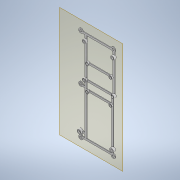
# Autodesk Inventor part: system_holder_plastic
Saved by Autodesk Inventor 2020 (Build 240168000, 168)
## iProperties
Created: 2020-01-14
Part Number: system_holder_plastic
Material: Generic
Document SubType Name: Modeling
Designer: erwin
Density: 1 g/cm^3
Appearance: Default
Author: erwin
Autodesk Inventor part; units mm, degrees
ref_plane "YZ Plane" through (0, 0, 0) normal (1, 0, 0) x (0, 1, 0)
ref_plane "XZ Plane" through (0, 0, 0) normal (0, 1, 0) x (-1, 0, 0)
ref_plane "XY Plane" through (0, 0, 0) normal (0, 0, 1) x (1, 0, 0)
ref_plane "Work Plane1" through (0, 0, 0) normal (0, 0, 1) x (1, 0, 0)
sketch "Sketch1" plane through (0, 0, 0) normal (0, 0, 1) x (1, 0, 0)
  circle A0 centre (-17, 43.4) radius 1.9 projected
  circle A1 centre (-17, 79.8) radius 1.9 projected
  circle A2 centre (39, -79.8) radius 1.9 projected
  circle A3 centre (-17, -79.8) radius 1.9 projected
  circle A4 centre (39, 79.8) radius 1.9 projected
  circle A5 centre (-17, 0) radius 1.9 projected
  circle A6 centre (39, 43.4) radius 1.9 construction
  arc A7 (-25.9799, 38.2) -> (-24, 40.1799) centre (-24.9899, 39.1899) ccw projected
  line L0 (-25.9799, 38.2) -> (-27.6, 38.2) projected
  line L1 (-27.6, 28.2) -> (-27.6, 38.2) projected
  line L2 (-27.6, 28.2) -> (-25.9799, 28.2) projected
  arc A8 (-24, 26.2201) -> (-25.9799, 28.2) centre (-24.9899, 27.2101) ccw projected
  line L3 (-24, 26.2201) -> (-24, 20.1799) projected
  arc A9 (-25.9799, 18.2) -> (-24, 20.1799) centre (-24.9899, 19.1899) ccw projected
  line L4 (-25.9799, 18.2) -> (-27.6, 18.2) projected
  line L5 (-27.6, -18.2) -> (-27.6, 18.2) projected
  line L6 (-27.6, -18.2) -> (-25.9799, -18.2) projected
  arc A10 (-24, -20.1799) -> (-25.9799, -18.2) centre (-24.9899, -19.1899) ccw projected
  line L7 (-24, -20.1799) -> (-24, -26.2201) projected
  arc A11 (-25.9799, -28.2) -> (-24, -26.2201) centre (-24.9899, -27.2101) ccw projected
  line L8 (-25.9799, -28.2) -> (-27.6, -28.2) projected
  line L9 (-27.6, -38.2) -> (-27.6, -28.2) projected
  line L10 (-27.6, -38.2) -> (-25.9799, -38.2) projected
  arc A12 (-24, -40.1799) -> (-25.9799, -38.2) centre (-24.9899, -39.1899) ccw projected
  line L11 (-24, -40.1799) -> (-24, -46.2201) projected
  arc A13 (-25.9799, -48.2) -> (-24, -46.2201) centre (-24.9899, -47.2101) ccw projected
  line L12 (-25.9799, -48.2) -> (-27.6, -48.2) projected
  line L13 (-27.6, -54.6) -> (-27.6, -48.2) projected
  line L14 (-36.9959, -54.6) -> (-27.6, -54.6) projected
  line L15 (-36.9945, -55.6) -> (-36.9959, -54.6) projected
  line L16 (-40.9945, -55.6) -> (-36.9945, -55.6) projected
  line L17 (-40.9959, -54.6) -> (-40.9945, -55.6) projected
  line L18 (-42.6, -54.6) -> (-40.9959, -54.6) projected
  arc A14 (-42.6, -54.6) -> (-42.6, -68.6) centre (-42.6, -61.6) ccw projected
  line L19 (-40.9761, -68.6) -> (-42.6, -68.6) projected
  line L20 (-40.9736, -67.6) -> (-40.9761, -68.6) projected
  line L21 (-36.9736, -67.6) -> (-40.9736, -67.6) projected
  line L22 (-36.9761, -68.6) -> (-36.9736, -67.6) projected
  line L23 (-27.6, -68.6) -> (-36.9761, -68.6) projected
  line L24 (-27.6, -75) -> (-27.6, -68.6) projected
  line L25 (-27.6, -75) -> (-25.9799, -75) projected
  arc A15 (-24, -76.9799) -> (-25.9799, -75) centre (-24.9899, -75.9899) ccw projected
  line L26 (-24, -76.9799) -> (-24, -86.8) projected
  line L27 (-24, -86.8) -> (46, -86.8) projected
  line L28 (46, -86.8) -> (46, -76.9799) projected
  arc A16 (47.9799, -75) -> (46, -76.9799) centre (46.9899, -75.9899) ccw projected
  line L29 (47.9799, -75) -> (49.6, -75) projected
  line L30 (49.6, -48.2) -> (49.6, -75) projected
  line L31 (49.6, -48.2) -> (47.9799, -48.2) projected
  arc A17 (46, -46.2201) -> (47.9799, -48.2) centre (46.9899, -47.2101) ccw projected
  line L32 (46, -46.2201) -> (46, -40.1799) projected
  arc A18 (47.9799, -38.2) -> (46, -40.1799) centre (46.9899, -39.1899) ccw projected
  line L33 (47.9799, -38.2) -> (49.6, -38.2) projected
  line L34 (49.6, -28.2) -> (49.6, -38.2) projected
  line L35 (49.6, -28.2) -> (47.9799, -28.2) projected
  arc A19 (46, -26.2201) -> (47.9799, -28.2) centre (46.9899, -27.2101) ccw projected
  line L36 (46, -26.2201) -> (46, -20.1799) projected
  arc A20 (47.9799, -18.2) -> (46, -20.1799) centre (46.9899, -19.1899) ccw projected
  line L37 (47.9799, -18.2) -> (49.6, -18.2) projected
  line L38 (49.6, 18.2) -> (49.6, -18.2) projected
  line L39 (49.6, 18.2) -> (47.9799, 18.2) projected
  arc A21 (46, 20.1799) -> (47.9799, 18.2) centre (46.9899, 19.1899) ccw projected
  line L40 (46, 20.1799) -> (46, 26.2201) projected
  arc A22 (47.9799, 28.2) -> (46, 26.2201) centre (46.9899, 27.2101) ccw projected
  line L41 (47.9799, 28.2) -> (49.6, 28.2) projected
  line L42 (49.6, 38.2) -> (49.6, 28.2) projected
  line L43 (49.6, 38.2) -> (47.9799, 38.2) projected
  arc A23 (46, 40.1799) -> (47.9799, 38.2) centre (46.9899, 39.1899) ccw projected
  line L44 (46, 40.1799) -> (46, 46.2201) projected
  arc A24 (47.9799, 48.2) -> (46, 46.2201) centre (46.9899, 47.2101) ccw projected
  line L45 (47.9799, 48.2) -> (49.6, 48.2) projected
  line L46 (49.6, 75) -> (49.6, 48.2) projected
  line L47 (49.6, 75) -> (47.9799, 75) projected
  arc A25 (46, 76.9799) -> (47.9799, 75) centre (46.9899, 75.9899) ccw projected
  line L48 (46, 76.9799) -> (46, 86.8) projected
  line L49 (46, 86.8) -> (-24, 86.8) projected
  line L50 (-24, 86.8) -> (-24, 76.9799) projected
  arc A26 (-25.9799, 75) -> (-24, 76.9799) centre (-24.9899, 75.9899) ccw projected
  line L51 (-25.9799, 75) -> (-27.6, 75) projected
  line L52 (-27.6, 68.6) -> (-27.6, 75) projected
  line L53 (-36.6, 68.6) -> (-27.6, 68.6) projected
  line L54 (-36.6, 67.6) -> (-36.6, 68.6) projected
  line L55 (-40.6, 67.6) -> (-36.6, 67.6) projected
  line L56 (-40.6, 68.6) -> (-40.6, 67.6) projected
  line L57 (-41.6163, 68.6) -> (-40.6, 68.6) projected
  arc A27 (-41.6163, 68.6) -> (-41.6163, 54.6) centre (-41.6163, 61.6) ccw projected
  line L58 (-40.6, 54.6) -> (-41.6163, 54.6) projected
  line L59 (-40.6, 55.6) -> (-40.6, 54.6) projected
  line L60 (-36.6, 55.6) -> (-40.6, 55.6) projected
  line L61 (-36.6, 54.6) -> (-36.6, 55.6) projected
  line L62 (-27.6, 54.6) -> (-36.6, 54.6) projected
  line L63 (-27.6, 48.2) -> (-27.6, 54.6) projected
  line L64 (-27.6, 48.2) -> (-25.9799, 48.2) projected
  arc A28 (-24, 46.2201) -> (-25.9799, 48.2) centre (-24.9899, 47.2101) ccw projected
  line L65 (-24, 46.2201) -> (-24, 40.1799) projected
  circle A29 centre (-17, 79.8) radius 1.7
  circle A30 centre (39, 79.8) radius 1.7
  circle A31 centre (-17, 0) radius 1.7
  circle A32 centre (-17, -79.8) radius 1.7
  circle A33 centre (39, -79.8) radius 1.7
  circle A34 centre (-17, 79.8) radius 3.7
  circle A35 centre (39, 79.8) radius 3.7
  circle A36 centre (-17, 0) radius 3.7
  circle A37 centre (-17, -79.8) radius 3.7
  circle A38 centre (39, -79.8) radius 3.7
  line L66 (-8.5, 11.3) -> (40.5, 11.3) construction
  line L67 (40.5, 11.3) -> (40.5, 69.3) construction
  line L68 (40.5, 69.3) -> (-8.5, 69.3) construction
  line L69 (-8.5, 69.3) -> (-8.5, 11.3) construction
  circle A39 centre (-8.5, 11.3) radius 3
  circle A40 centre (-8.5, 69.3) radius 3
  circle A41 centre (40.5, 11.3) radius 3
  circle A42 centre (40.5, 69.3) radius 3
  point P0 (0, 0)
  dimension "d0" = 0.2
  dimension "d1" = 0.2
  dimension "d2" = 0.2
  dimension "d3" = 0.2
  dimension "d4" = 0.2
  dimension "border" = 2
  dimension "d6" = 2
  dimension "d7" = 2
  dimension "d8" = 2
  dimension "d9" = 2
  dimension "d10" = 49
  dimension "d11" = 58
  dimension "d12" = 8.5
  dimension "d13" = 10.5
  dimension "pi_stand" = 6
  dimension "d15" = 6
  dimension "d16" = 6
  dimension "d17" = 6
  constraints: 14 centre point, 8 end point, 4 coincident, 2 parallel, 1 horizontal, 1 perpendicular
  measures "d0" radial gap between concentric circles of A1 A29
  measures "d1" radial gap between concentric circles of A4 A30
  measures "d2" radial gap between concentric circles of A31 A5
  measures "d3" radial gap between concentric circles of A32 A3
  measures "d4" radial gap between concentric circles of A33 A2
  measures "border" radial gap between concentric circles of A29 A34
  measures "d6" radial gap between concentric circles of A30 A35
  measures "d7" radial gap between concentric circles of A31 A36
  measures "d8" radial gap between concentric circles of A32 A37
  measures "d9" radial gap between concentric circles of A33 A38
  measures "d10" distance of L68.end L67.end
  measures "d11" distance of L67.end L66.end
  measures "d12" distance from line of A1.centre L69
  measures "d13" distance from line of A1.centre L68
  measures "pi_stand" diameter of A39
  measures "d15" diameter of A40
  measures "d16" diameter of A41
  measures "d17" diameter of A42
extrude "Extrusion1" add sketch "Sketch1" along normal blind 1 contours A1 | A2 | A3 | A4 | A5 | A34 | A35 | A36 | A37 | A38 | A39 | A40 | A41 | A42
sketch "Sketch2" plane through (0, 0, 0) normal (0, 0, 1) x (1, 0, 0)
  circle A0 centre (39, 79.8) radius 1.7 projected
  circle A1 centre (39, 79.8) radius 3.7 projected
  circle A2 centre (-17, 0) radius 1.7 projected
  circle A3 centre (-17, 0) radius 3.7 projected
  circle A4 centre (-17, -79.8) radius 1.7 projected
  circle A5 centre (-17, -79.8) radius 3.7 projected
  circle A6 centre (40.5, 69.3) radius 3 projected
  circle A7 centre (-8.5, 69.3) radius 3 projected
  circle A8 centre (40.5, 11.3) radius 3 projected
  circle A9 centre (39, -79.8) radius 1.7 projected
  circle A10 centre (39, -79.8) radius 3.7 projected
  circle A11 centre (-8.5, 11.3) radius 3 projected
  circle A12 centre (-17, 79.8) radius 1.7 projected
  circle A13 centre (-17, 79.8) radius 3.7 projected
  line L0 (38.3273, 69.3) -> (41.3273, 69.3)
  line L1 (41.3273, 69.3) -> (41.3273, 77.1843)
  line L2 (41.3273, 77.1843) -> (38.3273, 77.1843)
  line L3 (38.3273, 77.1843) -> (38.3273, 69.3)
  circle A14 centre (-17, 79.8) radius 3.7 projected
  line L4 (36.697, 80.4447) -> (-14.1465, 80.4447)
  line L5 (-14.1465, 80.4447) -> (-14.1465, 77.4447)
  line L6 (-14.1465, 77.4447) -> (36.697, 77.4447)
  line L7 (36.697, 77.4447) -> (36.697, 80.4447)
  line L8 (-9.8186, 79.1357) -> (-6.8186, 79.1357)
  line L9 (-6.8186, 79.1357) -> (-6.8186, 10.7535)
  line L10 (-6.8186, 10.7535) -> (-9.8186, 10.7535)
  line L11 (-9.8186, 10.7535) -> (-9.8186, 79.1357)
  circle A15 centre (40.5, 69.3) radius 3 projected
  line L12 (38.3273, 71.3686) -> (41.3273, 71.3686)
  line L13 (41.3273, 71.3686) -> (41.3273, 11.3)
  line L14 (41.3273, 11.3) -> (38.3273, 11.3)
  line L15 (38.3273, 11.3) -> (38.3273, 71.3686)
  line L16 (41.3273, 12.0577) -> (-9.8186, 12.0577)
  line L17 (-9.8186, 12.0577) -> (-9.8186, 9.0577)
  line L18 (-9.8186, 9.0577) -> (41.3273, 9.0577)
  line L19 (41.3273, 9.0577) -> (41.3273, 12.0577)
  line L20 (36.697, -79.8) -> (-17, -79.8)
  line L21 (-17, -79.8) -> (-17, -76.8)
  line L22 (-17, -76.8) -> (36.697, -76.8)
  line L23 (36.697, -76.8) -> (36.697, -79.8)
  line L24 (-6.8186, 9.8735) -> (-9.8186, 9.8735)
  line L25 (-9.8186, 9.8735) -> (-9.8186, -78.3)
  line L26 (-9.8186, -78.3) -> (-6.8186, -78.3)
  line L27 (-6.8186, -78.3) -> (-6.8186, 9.8735)
  circle A16 centre (-17, 0) radius 3.7 projected
  line L28 (-14.1465, -2.3553) -> (-8.0873, -2.3553)
  line L29 (-8.0873, -2.3553) -> (-8.0873, 0.6447)
  line L30 (-8.0873, 0.6447) -> (-14.1465, 0.6447)
  line L31 (-14.1465, 0.6447) -> (-14.1465, -2.3553)
  line L32 (39, -78.1) -> (36, -78.1)
  line L33 (36, -78.1) -> (36, 11.6)
  line L34 (36, 11.6) -> (39, 11.6)
  line L35 (39, 11.6) -> (39, -78.1)
  point P0 (0, 0)
  point P1 (-6.8186, 77.4447)
  point P2 (-9.8186, 77.4447)
  point P3 (-9.8186, 0.6447)
  point P4 (-13.3566, 0.6447)
  point P5 (-9.8186, -2.3553)
  point P6 (-9.8186, -76.8)
  point P7 (-17, -78.1)
  point P8 (-15.3, -79.8)
  point P9 (-6.8186, -76.8)
  point P10 (-6.8186, 9.0577)
  point P11 (38.3273, 12.0577)
  point P12 (-6.8186, 12.0577)
  point P13 (39, 9.0577)
  point P14 (36, 9.0577)
  point P15 (36, -76.8)
  point P16 (36.697, -78.1)
  dimension "d20" = 3
  dimension "d21" = 3
  dimension "d22" = 3
  dimension "d23" = 3
  dimension "d24" = 3
  dimension "d25" = 3
  dimension "d26" = 3
  dimension "d32" = 3
  constraints: 72 end point, 18 parallel, 9 horizontal, 9 perpendicular, 7 point on line, 1 vertical alignment, 7 other
  measures "d20" distance of L2.end L1.end
  measures "d21" distance of L5.end L4.end
  measures "d22" distance of L9.end L10.end
  measures "d23" distance of L17.end L16.end
  measures "d24" distance of L20.end L21.end
  measures "d25" distance of L26.end L25.end
  measures "d26" distance of L29.end L28.end
  measures "d32" distance of L33.end L34.end
move faces "Move1" translate (0, 0, 5) faces at (-8.843, 10.7311, 1) (-7.7224, 69.7238, 1) (39.666, 70.6672, 1) (41.4145, 10.596, 1)
extrude "Extrusion2" add sketch "Sketch2" along normal blind 1 contours L4 L7 L6 A1 | A1 L6 L9 L8 L11 A13 L4 | L1 A6 L3 A1 | A1 L3 L2 L1 | A13 L5 L4 | L1 L12 A6 | L9 A7 L11 L6 | L6 L11 L8 L9 | L12 L1 L0 L3 | L9 A7 L11 | L15 L0 L13 A6 | A6 L13 A8 L15 | L9 A11 L11 A7 | A8 L13 L16 L15 | L9 L16 L11 A11 | L16 L15 L34 A8 | A8 L34 L33 L18 A11 L16 | L16 L13 L14 L35 L34 L15 | A11 L18 L27 L24 L17 L10 L9 L16 | L9 L10 L11 L16 | L34 L15 L14 L35 L18 A8 | A8 L18 L33 L34 | L34 L35 L14 L15 | L35 A10 L23 L22 L33 L18 A8 | A8 L18 L35 | L19 L18 L35 L14 | L25 L18 L27 A11 | A11 L27 L22 L25 L28 L29 L30 | L35 L32 L23 A10 | L17 L24 L27 L18 | L30 L29 L28 L25 | L25 L28 A3 L30 | L23 L32 L33 A10 | A10 L33 L22 L23 | L27 L26 L25 L22 | L22 L33 A10 L20 A5 L25 L26 L27 | A10 L33 L32 L23 L20 | L20 A4 L21 L22 A5 picked at (-13.9926, 78.6822) picked at (-16.0323, -77.2895)
sketch "Sketch3" plane through (40.5, 11.3, 6) normal (0, 0, 1) x (1, 0, 0)
  circle A0 centre (0, 0) radius 3 projected
  circle A1 centre (-49, 0) radius 3 projected
  circle A2 centre (-49, 58) radius 3 projected
  circle A3 centre (0, 58) radius 3 projected
  point P0 (-40.5, -11.3)
  constraints: 4 coincident
hole "Hole1" at (40.5, 11.3, 6) at (-8.5, 11.3, 6) at (-8.5, 69.3, 6) at (40.5, 69.3, 6) direction (0, 0, -1) diameter 2 end through all
sketch "Sketch4" plane through (0, 0, 0) normal (0, 0, 1) x (1, 0, 0)
  circle A0 centre (-4.25, -4.7) radius 2.7443
  circle A1 centre (-4.25, 37.3) radius 2.7443
  circle A2 centre (36.25, 37.3) radius 2.7443
  circle A3 centre (36.25, -4.7) radius 2.7443
  circle A4 centre (36.25, -4.7) radius 1.35
  circle A5 centre (36.25, 37.3) radius 1.35
  circle A6 centre (-4.25, 37.3) radius 1.35
  circle A7 centre (-4.25, -4.7) radius 1.35
  line L0 (36.25, 37.3) -> (-4.25, 37.3) construction
  line L1 (-4.25, 37.3) -> (-4.25, -4.7) construction
  line L2 (-4.25, -4.7) -> (36.25, -4.7) construction
  line L3 (36.25, -4.7) -> (36.25, 37.3) construction
  circle A8 centre (40.5, 11.3) radius 1 construction
  circle A9 centre (40.5, 11.3) radius 3 construction
  circle A10 centre (-8.5, 11.3) radius 1 construction
  point P0 (0, 0)
  dimension "d40" = 17
  dimension "d41" = 42
  dimension "d42" = 40.5
  dimension "d43" = 4.25
  dimension "d44" = 4.25
  constraints: 8 centre point, 8 end point, 5 coincident, 2 parallel, 1 horizontal, 1 perpendicular
  measures "d41" distance of L2.end L0.start
  measures "d42" distance between parallel lines of L1 L3
  measures "d43" distance from line of A9.centre L3
  measures "d44" distance from line of L1 A10.centre
extrude "Extrusion3" add sketch "Sketch4" along normal blind 4 contours A0 | A1 | A2 | A3 | A4 | A5 | A6 | A7
sketch "Sketch5" plane through (36.25, 37.3, 4) normal (0, 0, 1) x (1, 0, 0)
  circle A0 centre (0, 0) radius 2.7443 construction
  circle A1 centre (-40.5, 0) radius 2.7443 construction
  circle A2 centre (-40.5, -42) radius 2.7443 construction
  circle A3 centre (0, -42) radius 2.7443 construction
  point P0 (-36.25, -37.3)
  constraints: 4 coincident
hole "Hole2" at (36.25, 37.3, 4) at (-4.25, 37.3, 4) at (-4.25, -4.7, 4) at (36.25, -4.7, 4) direction (0, 0, -1) diameter 2 end through all
sketch "Sketch6" plane through (36.25, -4.7, 4) normal (0, 0, 1) x (1, 0, 0)
  circle A0 centre (0, 0) radius 1 projected
  circle A1 centre (-40.5, 0) radius 1 projected
  line L0 (0, 0) -> (-40.5, 0)
  line L1 (-20.25, 0) -> (-20.25, 27.3272) construction
  line L2 (2.75, 21.0276) -> (-43.25, 21.0276)
  line L3 (-43.25, 21.0276) -> (-43.25, 10.7425)
  line L4 (-43.25, 10.7425) -> (2.75, 10.7425)
  line L5 (2.75, 10.7425) -> (2.75, 21.0276)
  line L6 (2.75, 21.0276) -> (-43.25, 10.7425) construction
  line L7 (-43.25, 21.0276) -> (2.75, 10.7425) construction
  point P0 (-36.25, 4.7)
  point P1 (-20.25, 15.885)
  dimension "d54" = 46
  constraints: 16 end point, 3 midpoint, 2 horizontal, 2 parallel, 1 perpendicular, 1 point on line, 1 vertical
  measures "d54" distance of L4.end L3.end
extrude "Extrusion4" cut sketch "Sketch6" along normal blind 4 contours L5 L4 L3 L2
sketch "Sketch7" plane through (0, 0, 0) normal (0, 0, -1) x (-1, 0, 0)
  circle A0 centre (4.25, -4.7) radius 2.7443 projected
  line L0 (-35.0313, -5.2506) -> (3.0124, -5.2506)
  line L1 (3.0124, -5.2506) -> (3.0124, -2.2506)
  line L2 (3.0124, -2.2506) -> (-35.0313, -2.2506)
  line L3 (-35.0313, -2.2506) -> (-35.0313, -5.2506)
  line L4 (-34.4738, 35.8768) -> (3.25, 35.8768)
  line L5 (3.25, 35.8768) -> (3.25, 38.8768)
  line L6 (3.25, 38.8768) -> (-34.4738, 38.8768)
  line L7 (-34.4738, 38.8768) -> (-34.4738, 35.8768)
  point P0 (0, 0)
  dimension "d57" = 3
  dimension "d58" = 3
  constraints: 16 end point, 4 parallel, 2 horizontal, 2 perpendicular, 2 other
  measures "d57" distance of L1.end L0.end
  measures "d58" distance of L5.end L4.end
extrude "Extrusion5" add sketch "Sketch7" against normal blind 1 contours L1 L0 A0 | A0 L0 L3 L2 | L7 L6 L5 L4 picked at (2.8459, -3.3589)
sketch "Sketch8" plane through (0, 0, 0) normal (0, 0, -1) x (-1, 0, 0)
  line L0 (8.3128, 36.1371) -> (5.4091, 36.1371)
  line L1 (5.4091, 36.1371) -> (5.4091, 39.1371)
  line L2 (5.4091, 39.1371) -> (8.3128, 39.1371)
  line L3 (8.3128, 39.1371) -> (8.3128, 36.1371)
  line L4 (5.4091, -5.2304) -> (7.8286, -5.2304)
  line L5 (7.8286, -5.2304) -> (7.8286, -2.2304)
  line L6 (7.8286, -2.2304) -> (5.4091, -2.2304)
  line L7 (5.4091, -2.2304) -> (5.4091, -5.2304)
  point P0 (0, 0)
  dimension "d61" = 3
  dimension "d62" = 3
  constraints: 16 end point, 4 parallel, 2 horizontal, 2 perpendicular
  measures "d61" distance of L0.end L1.end
  measures "d62" distance of L5.end L4.end
extrude "Extrusion6" add sketch "Sketch8" against normal blind 1
sketch "Sketch9" plane through (0, 0, 0) normal (0, 0, 1) x (1, 0, 0)
  circle A0 centre (39, -79.8) radius 1.7 construction
  circle A1 centre (-17, -79.8) radius 1.7 construction
  line L0 (39, -79.8) -> (-17, -79.8) construction
  line L1 (-17, -79.8) -> (-17, -69.8) construction
  line L2 (-17, -69.8) -> (39, -69.8) construction
  line L3 (39, -69.8) -> (39, -79.8) construction
  circle A2 centre (39, -69.8) radius 3.4
  circle A3 centre (-17, -69.8) radius 3.4
  point P0 (0, 0)
  dimension "d65" = 10
  dimension "d66" = 6.8
  dimension "d67" = 6.8
  constraints: 8 end point, 2 centre point, 2 coincident, 2 parallel, 1 horizontal, 1 perpendicular
  measures "d65" distance of L0.end L1.end
  measures "d66" diameter of A2
  measures "d67" diameter of A3
extrude "Extrusion7" add sketch "Sketch9" along normal blind 4
sketch "Sketch10" plane through (0, 0, 0) normal (0, 0, -1) x (-1, 0, 0)
  line L0 (17.2808, -68.6854) -> (7.98, -68.6854)
  line L1 (7.98, -68.6854) -> (7.98, -71.6854)
  line L2 (7.98, -71.6854) -> (17.2808, -71.6854)
  line L3 (17.2808, -71.6854) -> (17.2808, -68.6854)
  line L4 (17.9548, -70.1854) -> (14.9548, -70.1854)
  line L5 (14.9548, -70.1854) -> (14.9548, -78.1854)
  line L6 (14.9548, -78.1854) -> (17.9548, -78.1854)
  line L7 (17.9548, -78.1854) -> (17.9548, -70.1854)
  point P0 (0, 0)
  point P1 (14.9548, -71.6854)
  point P2 (17.2808, -70.1854)
  dimension "d70" = 3
  dimension "d71" = 3
  dimension "d72" = 8
  constraints: 16 end point, 4 parallel, 2 horizontal, 2 perpendicular
  measures "d70" distance of L1.end L0.end
  measures "d71" distance of L6.end L5.end
  measures "d72" distance of L5.end L4.end
extrude "Extrusion8" add sketch "Sketch10" against normal blind 1
sketch "Sketch11" plane through (39, -69.8, 4) normal (0, 0, 1) x (1, 0, 0)
  circle A0 centre (0, 0) radius 3.4 projected
  circle A1 centre (-56, 0) radius 3.4 projected
  point P0 (-39, 69.8)
  constraints: 2 coincident
hole "Hole3" at (39, -69.8, 4) at (-17, -69.8, 4) direction (0, 0, -1) diameter 2 end through all
move faces "Move2" translate (0, 0, -1) faces at (-2.1162, -4.9591, 4) (-2.1162, 37.0409, 4) (38.3838, 37.0409, 4) (38.3838, -4.9591, 4) (-6.8309, 12.0431, 4) (38.5603, 11.642, 4)
move faces "Move3" translate (0, 0, -2) faces at (-10.8018, 69.5795, 6) (38.1982, 69.5795, 6) (39.1691, 11.2598, 6) (-7.1691, 11.2598, 6)
chamfer "Chamfer1" distance 1 angle 45 10 edges at (-8.5, 70.3, 4) (40.5, 70.3, 4) (36.25, 38.3, 3) (-4.25, 38.3, 3) (-8.5, 12.3, 4) (-4.25, -3.7, 3) (36.25, -3.7, 3) (40.5, 12.3, 4) (39, -68.8, 4) (-17, -68.8, 4)
equation "\"d1\" = d0"
equation "\"d2\" = d0"
equation "\"d3\" = d0"
equation "\"d4\" = d0"
equation "\"d6\" = border"
equation "\"d7\" = border"
equation "\"d8\" = border"
equation "\"d9\" = border"
equation "\"d15\" = pi_stand"
equation "\"d16\" = pi_stand"
equation "\"d17\" = pi_stand"
equation "\"d43\" = d44"
equation "\"d67\" = d66"
body "Solid1"
